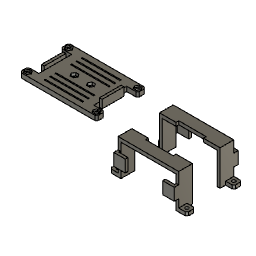
Bbox_lite_mount (Autodesk Fusion 360 design; units mm, degrees)
Autodesk Fusion 360 part; units mm, degrees
note: some values were not read from the file. Set by a fixed rule: which face or edge a step refers to.
sketch "Sketch1" plane through (0, 0, 0) normal (0, 0, 1) x (1, 0, 0)
  line L0 (0, 0) -> (100.25, 0)
  line L1 (100.25, 0) -> (100.25, -89.65)
  line L2 (100.25, -89.65) -> (0, -89.65)
  line L3 (0, -89.65) -> (0, 0)
  line L4 (100.25, 0) -> (105.25, 0)
  line L5 (105.25, 0) -> (105.25, -15)
  line L6 (105.25, -15) -> (100.25, -15)
  line L7 (100.25, -15) -> (100.25, 0)
  line L8 (105.25, 0) -> (120.25, 0)
  line L9 (120.25, 0) -> (120.25, -15)
  line L10 (120.25, -15) -> (105.25, -15)
  line L11 (105.25, -15) -> (105.25, 0)
  line L12 (100.25, -89.65) -> (105.25, -89.65)
  line L13 (105.25, -89.65) -> (105.25, -74.65)
  line L14 (105.25, -74.65) -> (100.25, -74.65)
  line L15 (100.25, -74.65) -> (100.25, -89.65)
  line L16 (105.25, -89.65) -> (120.25, -89.65)
  line L17 (120.25, -89.65) -> (120.25, -74.65)
  line L18 (120.25, -74.65) -> (105.25, -74.65)
  line L19 (105.25, -74.65) -> (105.25, -89.65)
  line L20 (0, 0) -> (-5, 0)
  line L21 (-5, 0) -> (-5, -15)
  line L22 (-5, -15) -> (0, -15)
  line L23 (0, -15) -> (0, 0)
  line L24 (0, -89.65) -> (-5, -89.65)
  line L25 (-5, -89.65) -> (-5, -74.65)
  line L26 (-5, -74.65) -> (0, -74.65)
  line L27 (0, -74.65) -> (0, -89.65)
  line L28 (-5, -74.65) -> (-19.7343, -74.65)
  line L29 (-19.7343, -74.65) -> (-19.7343, -89.65)
  line L30 (-19.7343, -89.65) -> (-5, -89.65)
  line L31 (-5, -89.65) -> (-5, -74.65)
  line L32 (-5, -15) -> (-20, -15)
  line L33 (-20, -15) -> (-20, 0)
  line L34 (-20, 0) -> (-5, 0)
  line L35 (-5, 0) -> (-5, -15)
  line L36 (105.25, -25) -> (100.25, -25)
  line L37 (100.25, -25) -> (100.25, -64.65)
  line L38 (100.25, -64.65) -> (105.25, -64.65)
  line L39 (105.25, -64.65) -> (105.25, -25)
  line L40 (0, -25) -> (0, -65)
  line L41 (-5, -25) -> (0, -25)
  line L42 (0, -25) -> (0, -64.65)
  line L43 (0, -64.65) -> (-5, -64.65)
  line L44 (-5, -64.65) -> (-5, -25)
  line L45 (109.6301, -12.6251) -> (115.6285, -12.7644)
  line L46 (115.6285, -12.7644) -> (118.7484, -7.6394)
  line L47 (118.7484, -7.6394) -> (115.8699, -2.3749)
  line L48 (115.8699, -2.3749) -> (109.8715, -2.2356)
  line L49 (109.8715, -2.2356) -> (106.7516, -7.3606)
  line L50 (106.7516, -7.3606) -> (109.6301, -12.6251)
  circle A0 centre (112.75, -7.5) radius 3.05
  line L51 (109.75, -87.3462) -> (115.75, -87.3462)
  line L52 (115.75, -87.3462) -> (118.75, -82.15)
  line L53 (118.75, -82.15) -> (115.75, -76.9538)
  line L54 (115.75, -76.9538) -> (109.75, -76.9538)
  line L55 (109.75, -76.9538) -> (106.75, -82.15)
  line L56 (106.75, -82.15) -> (109.75, -87.3462)
  line L57 (109.75, -87.3462) -> (115.75, -87.3462) construction
  circle A1 centre (112.75, -82.15) radius 3.05
  line L58 (-15.2555, -87.3338) -> (-9.2556, -87.3584)
  line L59 (-9.2556, -87.3584) -> (-6.2344, -82.1745)
  line L60 (-6.2344, -82.1745) -> (-9.2131, -76.9662)
  line L61 (-9.2131, -76.9662) -> (-15.213, -76.9416)
  line L62 (-15.213, -76.9416) -> (-18.2343, -82.1255)
  line L63 (-18.2343, -82.1255) -> (-15.2555, -87.3338)
  circle A2 centre (-12.2343, -82.15) radius 3.05
  line L64 (-15.5, -12.6962) -> (-9.5, -12.6962)
  line L65 (-9.5, -12.6962) -> (-6.5, -7.5)
  line L66 (-6.5, -7.5) -> (-9.5, -2.3038)
  line L67 (-9.5, -2.3038) -> (-15.5, -2.3038)
  line L68 (-15.5, -2.3038) -> (-18.5, -7.5)
  line L69 (-18.5, -7.5) -> (-15.5, -12.6962)
  line L70 (-15.5, -12.6962) -> (-15.4999, -12.6962) construction
  circle A3 centre (-12.5, -7.5) radius 3.05
  line L71 (15, -10) -> (85, -10)
  line L72 (85, -10) -> (85, -12)
  line L73 (85, -12) -> (15, -12)
  line L74 (15, -12) -> (15, -10)
  line L75 (15, -20) -> (85, -20)
  line L76 (85, -20) -> (85, -22)
  line L77 (85, -22) -> (15, -22)
  line L78 (15, -22) -> (15, -20)
  line L79 (15, -30) -> (85, -30)
  line L80 (85, -30) -> (85, -32)
  line L81 (85, -32) -> (15, -32)
  line L82 (15, -32) -> (15, -30)
  line L83 (15, -80) -> (85, -80)
  line L84 (85, -80) -> (85, -78)
  line L85 (85, -78) -> (15, -78)
  line L86 (15, -78) -> (15, -80)
  line L87 (15, -70) -> (85, -70)
  line L88 (85, -70) -> (85, -68)
  line L89 (85, -68) -> (15, -68)
  line L90 (15, -68) -> (15, -70)
  line L91 (15, -60) -> (85, -60)
  line L92 (85, -60) -> (85, -58)
  line L93 (85, -58) -> (15, -58)
  line L94 (15, -58) -> (15, -60)
  line L95 (50.125, -44.825) -> (0, -45)
  line L96 (50.125, -44.825) -> (100.25, -44.825)
  line L97 (32.125, -39.6812) -> (29.125, -44.8774)
  line L98 (29.125, -44.8774) -> (32.125, -50.0735)
  line L99 (32.125, -50.0735) -> (38.125, -50.0735)
  line L100 (38.125, -50.0735) -> (41.125, -44.8774)
  line L101 (41.125, -44.8774) -> (38.125, -39.6812)
  line L102 (38.125, -39.6812) -> (32.125, -39.6812)
  line L103 (62.125, -50.0212) -> (68.125, -50.0212)
  line L104 (68.125, -50.0212) -> (71.125, -44.825)
  line L105 (71.125, -44.825) -> (68.125, -39.6288)
  line L106 (68.125, -39.6288) -> (62.125, -39.6288)
  line L107 (62.125, -39.6288) -> (59.125, -44.825)
  line L108 (59.125, -44.825) -> (62.125, -50.0212)
  circle A4 centre (35.125, -44.8774) radius 3.05
  circle A5 centre (65.125, -44.825) radius 3.05
  point P0 (112.75, -7.5)
  point P1 (112.75, -82.15)
  point P2 (-12.2343, -82.15)
  point P3 (-12.5, -7.5)
  point P4 (35.125, -44.8774)
  point P5 (65.125, -44.825)
  dimension "d1" = 100.25
  dimension "d2" = 89.65
  dimension "d3" = 5
  dimension "d4" = 15
  dimension "d5" = 15
  dimension "d6" = 15
  dimension "d7" = 5
  dimension "d8" = 15
  dimension "d9" = 15
  dimension "d10" = 15
  dimension "d11" = 5
  dimension "d12" = 15
  dimension "d13" = 15
  dimension "d18" = 39.65
  dimension "d19" = 6
  dimension "d20" = 7.5
  dimension "d21" = 7.5
  dimension "d22" = 6.1
  dimension "d23" = 6
  dimension "d24" = 0
  dimension "d25" = 7.5
  dimension "d26" = 7.5
  dimension "d27" = 6.1
  dimension "d28" = 6
  dimension "d29" = 7.5
  dimension "d30" = 7.5
  dimension "d31" = 6.1
  dimension "d32" = 6
  dimension "d33" = 0
  dimension "d35" = 7.5
  dimension "d36" = 7.5
  dimension "d37" = 6.1
  dimension "d38" = 70
  dimension "d39" = 2
  dimension "d40" = 70
  dimension "d41" = 2
  dimension "d42" = 70
  dimension "d43" = 2
  dimension "d44" = 70
  dimension "d45" = 2
  dimension "d46" = 70
  dimension "d47" = 2
  dimension "d48" = 70
  dimension "d49" = 2
  dimension "d50" = 50.125
  dimension "d51" = 44.825
  dimension "d52" = 6
  dimension "d53" = 15
  dimension "d56" = 15
  dimension "d57" = 6.1
  dimension "d58" = 6.1
  constraint horizontal L0
  constraint vertical L1
  constraint horizontal L2
  constraint vertical L3
  constraint coincident L0.start L3.end
  constraint horizontal L4
  constraint vertical L5
  constraint horizontal L6
  constraint vertical L7
  constraint horizontal L8
  constraint vertical L9
  constraint horizontal L10
  constraint vertical L11
  constraint horizontal L12
  constraint vertical L13
  constraint horizontal L14
  constraint vertical L15
  constraint horizontal L16
  constraint vertical L17
  constraint horizontal L18
  constraint vertical L19
  constraint horizontal L20
  constraint vertical L21
  constraint horizontal L22
  constraint vertical L23
  constraint horizontal L24
  constraint vertical L25
  constraint horizontal L26
  constraint vertical L27
  constraint horizontal L28
  constraint vertical L29
  constraint horizontal L30
  constraint vertical L31
  constraint horizontal L32
  constraint vertical L33
  constraint horizontal L34
  constraint vertical L35
  constraint horizontal L36
  constraint vertical L37
  constraint horizontal L38
  constraint vertical L39
  constraint coincident L1 L37.end
  constraint vertical L40
  constraint coincident L3 L40.end
  constraint horizontal L41
  constraint vertical L42
  constraint horizontal L43
  constraint vertical L44
  constraint coincident P0 A0.centre
  constraint horizontal L57
  constraint coincident P1 A1.centre
  constraint coincident P2 A2.centre
  constraint horizontal L70
  constraint coincident P3 A3.centre
  constraint horizontal L71
  constraint vertical L72
  constraint horizontal L73
  constraint vertical L74
  constraint horizontal L75
  constraint vertical L76
  constraint horizontal L77
  constraint vertical L78
  constraint horizontal L79
  constraint vertical L80
  constraint horizontal L81
  constraint vertical L82
  constraint horizontal L83
  constraint vertical L84
  constraint horizontal L85
  constraint vertical L86
  constraint horizontal L87
  constraint vertical L88
  constraint horizontal L89
  constraint vertical L90
  constraint horizontal L91
  constraint vertical L92
  constraint horizontal L93
  constraint vertical L94
  constraint midpoint L40 L95.end
  constraint midpoint L37 L96.end
  constraint perpendicular L37 L96
  constraint coincident L95 P4
  constraint coincident L96 P5
  constraint coincident P4 A4.centre
  constraint coincident P5 A5.centre
  measures "d1" distance of L0.start L0.end
  measures "d2" distance of L0.start L2.end
  measures "d3" distance of L0.end L4.end
  measures "d4" distance of L0.end L6.end
  measures "d5" distance of L4.end L8.end
  measures "d6" distance of L4.end L5.end
  measures "d7" distance of L1.end L12.end
  measures "d8" distance of L1.end L14.end
  measures "d9" distance of L12.end L16.end
  measures "d10" distance of L12.end L13.end
  measures "d11" distance of L2.end L24.end
  measures "d12" distance of L2.end L26.end
  measures "d13" distance of L25.end L24.end
  measures "d18" distance of L41.start L43.end
  measures "d19" distance of L45.start L45.end
  measures "d20" distance of L10 P0
  measures "d21" distance of L9 P0
  measures "d22" diameter of A0
  measures "d23" distance of L51.start L51.end
  measures "d24" angle of L51 L57
  measures "d25" distance of L17 P1
  measures "d26" distance of L16 P1
  measures "d27" diameter of A1
  measures "d28" distance of L58.start L58.end
  measures "d29" distance of L29 P2
  measures "d30" distance of L30 P2
  measures "d31" diameter of A2
  measures "d32" distance of L64.start L64.end
  measures "d33" angle of L64 L70
  measures "d35" distance of L35 P3
  measures "d36" distance of L32 P3
  measures "d37" diameter of A3
  measures "d38" distance of L71.start L71.end
  measures "d39" distance of L71.start L73.end
  measures "d40" distance of L75.start L75.end
  measures "d41" distance of L75.start L77.end
  measures "d42" distance of L79.start L79.end
  measures "d43" distance of L79.start L81.end
  measures "d44" distance of L83.start L83.end
  measures "d45" distance of L83.start L85.end
  measures "d46" distance of L87.start L87.end
  measures "d47" distance of L87.start L89.end
  measures "d48" distance of L91.start L91.end
  measures "d49" distance of L91.start L93.end
  measures "d50" distance of L1 L95.start
  measures "d51" distance of L2 L95.start
  measures "d52" distance of L97.start L101.end
  measures "d53" horizontal distance of L95.start P4
  measures "d56" distance of L95.start P5
  measures "d57" diameter of A4
  measures "d58" diameter of A5
extrude "Extrude1" add sketch "Sketch1" along normal blind 8.35 contours L0 L1 L3 L7 L23 L37 L40 L42 L95 L96 L97 L98 L101 L102 L105 L106 L107 | L3 L20 L21 L22 L23 L35 | L1 L4 L5 L6 L7 L11 | L21 L32 L33 L34 L35 | L5 L8 L9 L10 L11 | L1 L2 L3 L15 L27 L37 L40 L42 L95 L96 L98 L99 L100 L101 L103 L104 L108 | L1 L12 L13 L14 L15 L19 | L3 L24 L25 L26 L27 L31 | L13 L16 L17 L18 L19 | L25 L28 L29 L30 L31 makes body 1
extrude "Extrude2" add sketch "Sketch1" along normal blind 15 contours L3 L40 L41 L42 L43 L44 | L1 L36 L37 L38 L39 bodies 1
extrude "Extrude3" add sketch "Sketch1" along normal blind 5.75 contours L45 L46 L47 L48 L49 L50 | L51 L52 L53 L54 L55 L56 | L58 L59 L60 L61 L62 L63 | L64 L65 L66 L67 L68 L69 bodies 1
extrude "Extrude4" add sketch "Sketch1" along normal blind 3.25 contours L95 L97 L98 L101 L102 A4 | L95 L98 L99 L100 L101 A4 | L96 L103 L104 L108 A5 | L96 L105 L106 L107 A5 bodies 1
chamfer "Chamfer1" distance 3 angle 45 8 edges at (120.25, -89.65, 4.175) (120.25, -74.65, 4.175) (120.25, -15, 4.175) (120.25, 0, 4.175) (-19.7343, -89.65, 4.175) (-19.7343, -74.65, 4.175) (-20, -15, 4.175) (-20, 0, 4.175) on bodies 1
sketch "Sketch2" plane through (0, 0, 0) normal (0, 0, 1) x (1, 0, 0)
  line L0 (175, 0) -> (275.25, 0)
  line L1 (275.25, 0) -> (275.25, -25)
  line L2 (275.25, -25) -> (175, -25)
  line L3 (175, -25) -> (175, 0)
  line L4 (175, 0) -> (170, 0)
  line L5 (170, 0) -> (170, -25)
  line L6 (170, -25) -> (175, -25)
  line L7 (175, -25) -> (175, 0)
  line L8 (275.25, 0) -> (280.25, 0)
  line L9 (280.25, 0) -> (280.25, -25)
  line L10 (280.25, -25) -> (275.25, -25)
  line L11 (275.25, -25) -> (275.25, 0)
  line L12 (200, -25) -> (250, -25)
  line L13 (250, -25) -> (250, -20)
  line L14 (250, -20) -> (200, -20)
  line L15 (200, -20) -> (200, -25)
  dimension "d68" = 100.25
  dimension "d69" = 25
  dimension "d70" = 5
  dimension "d71" = 5
  constraint horizontal L0
  constraint vertical L1
  constraint horizontal L2
  constraint vertical L3
  constraint horizontal L4
  constraint vertical L5
  constraint horizontal L6
  constraint vertical L7
  constraint horizontal L8
  constraint vertical L9
  constraint horizontal L10
  constraint vertical L11
  constraint horizontal L12
  constraint vertical L13
  constraint horizontal L14
  constraint vertical L15
  constraint coincident L2 L12.start
  measures "d68" distance of L0.start L0.end
  measures "d69" distance of L0.start L2.end
  measures "d70" distance of L0.start L4.end
  measures "d71" distance of L0.end L8.end
extrude "Extrude5" add sketch "Sketch2" along normal blind 6.35 separate body contours L0 L1 L2 L3 L7 L11 L13 L14 L15 | L3 L4 L5 L6 L7 | L1 L8 L9 L10 L11 makes body 2
extrude "Extrude6" add sketch "Sketch2" against normal blind 57.55 contours L3 L4 L5 L6 L7 | L1 L8 L9 L10 L11 bodies 2
sketch "Sketch3" plane through (280.25, 0, 0) normal (1, 0, 0) x (0, 1, 0)
  line L0 (0, -57.55) -> (0, 6.35)
  line L1 (0, 6.35) -> (-25, 6.35)
  line L2 (-25, 6.35) -> (-25, -57.55)
  line L3 (-25, -57.55) -> (0, -57.55)
  line L4 (0, -57.55) -> (-15, -57.55)
  line L5 (-15, -57.55) -> (-15, -51.2)
  line L6 (-15, -51.2) -> (0, -51.2)
  line L7 (0, -51.2) -> (0, -57.55)
  dimension "d76" = 15
  dimension "d77" = 6.35
  constraint horizontal L4
  constraint vertical L5
  constraint horizontal L6
  constraint vertical L7
  constraint coincident L0.start L3.end
  measures "d76" distance of L0.start L4.end
  measures "d77" distance of L0.start L6.end
extrude "Extrude7" add sketch "Sketch3" along normal blind 15 contours L0 L3 L4 L5 L6 L7 bodies 2
sketch "Sketch4" plane through (170, 0, 0) normal (-1, 0, 0) x (0, -1, 0)
  line L0 (25, -57.55) -> (25, 6.35)
  line L1 (25, 6.35) -> (0, 6.35)
  line L2 (0, 6.35) -> (0, -57.55)
  line L3 (0, -57.55) -> (25, -57.55)
  line L4 (0, -57.55) -> (15, -57.55)
  line L5 (15, -57.55) -> (15, -51.2)
  line L6 (15, -51.2) -> (0, -51.2)
  line L7 (0, -51.2) -> (0, -57.55)
  dimension "d80" = 15
  dimension "d81" = 6.35
  constraint horizontal L4
  constraint vertical L5
  constraint horizontal L6
  constraint vertical L7
  constraint coincident L2.end L3.start
  measures "d80" distance of L2.end L4.end
  measures "d81" distance of L2.end L6.end
extrude "Extrude8" add sketch "Sketch4" along normal blind 15 contours L2 L3 L4 L5 L6 L7 bodies 2
sketch "Sketch5" plane through (0, 0, -51.2) normal (0, 0, 1) x (-1, 0, 0)
  line L0 (-280.25, 0) -> (-280.25, 15)
  line L1 (-280.25, 15) -> (-295.25, 15)
  line L2 (-295.25, 15) -> (-295.25, 0)
  line L3 (-295.25, 0) -> (-280.25, 0)
  line L4 (-284.7018, 2.332) -> (-281.7503, 7.5558)
  line L5 (-281.7503, 7.5558) -> (-284.7985, 12.7238)
  line L6 (-284.7985, 12.7238) -> (-290.7982, 12.668)
  line L7 (-290.7982, 12.668) -> (-293.7497, 7.4442)
  line L8 (-293.7497, 7.4442) -> (-290.7015, 2.2762)
  line L9 (-290.7015, 2.2762) -> (-284.7018, 2.332)
  circle A0 centre (-287.75, 7.5) radius 3.05
  point P0 (-287.75, 7.5)
  dimension "d84" = 6
  dimension "d85" = 7.5
  dimension "d86" = 7.5
  dimension "d87" = 6.1
  constraint coincident P0 A0.centre
  measures "d84" distance of L4.start L8.end
  measures "d85" distance of L3 P0
  measures "d86" distance of L2 P0
  measures "d87" diameter of A0
sketch "Sketch6" plane through (0, 0, -57.55) normal (0, 0, -1) x (1, 0, 0)
  line L0 (280.25, 25) -> (275.25, 25)
  line L1 (275.25, 25) -> (275.25, 0)
  line L2 (275.25, 0) -> (295.25, 0)
  line L3 (295.25, 0) -> (295.25, 15)
  line L4 (295.25, 15) -> (280.25, 15)
  line L5 (280.25, 15) -> (280.25, 25)
  circle A0 centre (287.75, 7.5) radius 3.05
  line L6 (290.7982, 12.668) -> (293.7497, 7.4442)
  line L7 (293.7497, 7.4442) -> (290.7015, 2.2762)
  line L8 (290.7015, 2.2762) -> (284.7018, 2.332)
  line L9 (284.7018, 2.332) -> (281.7503, 7.5558)
  line L10 (281.7503, 7.5558) -> (284.7985, 12.7238)
  line L11 (284.7985, 12.7238) -> (290.7982, 12.668)
  point P0 (287.75, 7.5)
sketch "Sketch7" plane through (0, 0, -51.2) normal (0, 0, 1) x (-1, 0, 0)
  line L0 (-170, 15) -> (-170, 0)
  line L1 (-170, 0) -> (-155, 0)
  line L2 (-155, 0) -> (-155, 15)
  line L3 (-155, 15) -> (-170, 15)
  line L4 (-159.4638, 2.3249) -> (-156.5001, 7.5419)
  line L5 (-156.5001, 7.5419) -> (-159.5363, 12.717)
  line L6 (-159.5363, 12.717) -> (-165.5362, 12.6751)
  line L7 (-165.5362, 12.6751) -> (-168.4999, 7.4581)
  line L8 (-168.4999, 7.4581) -> (-165.4637, 2.283)
  line L9 (-165.4637, 2.283) -> (-159.4638, 2.3249)
  circle A0 centre (-162.5, 7.5) radius 3.05
  point P0 (-162.5, 7.5)
  dimension "d88" = 6
  dimension "d89" = 7.5
  dimension "d90" = 7.5
  dimension "d91" = 6.1
  constraint coincident P0 A0.centre
  measures "d88" distance of L4.start L8.end
  measures "d89" distance of L1 P0
  measures "d90" distance of L2 P0
  measures "d91" diameter of A0
sketch "Sketch8" plane through (0, 0, -57.55) normal (0, 0, -1) x (1, 0, 0)
  line L0 (175, 0) -> (175, 25)
  line L1 (175, 25) -> (170, 25)
  line L2 (170, 25) -> (170, 15)
  line L3 (170, 15) -> (155, 15)
  line L4 (155, 15) -> (155, 0)
  line L5 (155, 0) -> (175, 0)
  circle A0 centre (162.5, 7.5) radius 3.05
  line L6 (159.4638, 2.3249) -> (156.5001, 7.5419)
  line L7 (165.4637, 2.283) -> (159.4638, 2.3249)
  line L8 (168.4999, 7.4581) -> (165.4637, 2.283)
  line L9 (165.5362, 12.6751) -> (168.4999, 7.4581)
  line L10 (159.5363, 12.717) -> (165.5362, 12.6751)
  line L11 (156.5001, 7.5419) -> (159.5363, 12.717)
  point P0 (162.5, 7.5)
chamfer "Chamfer2" distance 3 angle 45 4 edges at (295.25, -15, -54.375) (295.25, 0, -54.375) (155, -15, -54.375) (155, 0, -54.375) on bodies 2
extrude "Extrude9" cut sketch "Sketch8" sketch "Sketch6" against normal blind 2.5 contours L6 L7 L8 L9 L10 L11 of sketch 2 contours L6 L7 L8 L9 L10 L11 bodies 2
extrude "Extrude10" cut 2 faces at (163.1505, -6.9273, -57.55) (288.2946, -8.1401, -57.55) along direction (0, 0, 1) blind 6.35 on bodies 2 bodies 2
sketch "Sketch9" plane through (175, 0, 0) normal (1, 0, 0) x (0, 1, 0)
  line L0 (0, 0) -> (-25, 0)
  line L1 (-25, 0) -> (-25, -57.55)
  line L2 (-25, -57.55) -> (0, -57.55)
  line L3 (0, -57.55) -> (0, 0)
  line L4 (-15, -51.2) -> (0, -51.2)
  line L5 (-15, -51.2) -> (-15, -57.55)
sketch "Sketch10" plane through (275.25, 0, 0) normal (-1, 0, 0) x (0, -1, 0)
  line L0 (25, 0) -> (0, 0)
  line L1 (0, 0) -> (0, -57.55)
  line L2 (0, -57.55) -> (25, -57.55)
  line L3 (25, -57.55) -> (25, 0)
  line L4 (0, -51.2) -> (15, -51.2)
  line L5 (15, -57.55) -> (15, -51.2)
sketch "Sketch11" plane through (0, 0, 0) normal (0, 1, 0) x (-1, 0, 0)
  line L0 (-158, -57.55) -> (-158, -51.2)
  line L1 (-158, -51.2) -> (-170, -51.2)
  line L2 (-170, -51.2) -> (-170, 6.35)
  line L3 (-170, 6.35) -> (-280.25, 6.35)
  line L4 (-280.25, 6.35) -> (-280.25, -51.2)
  line L5 (-280.25, -51.2) -> (-292.25, -51.2)
  line L6 (-292.25, -51.2) -> (-292.25, -57.55)
  line L7 (-292.25, -57.55) -> (-275.25, -57.55)
  line L8 (-275.25, -57.55) -> (-275.25, 0)
  line L9 (-275.25, 0) -> (-175, 0)
  line L10 (-175, 0) -> (-175, -57.55)
  line L11 (-175, -57.55) -> (-158, -57.55)
  line L12 (-280.25, -14.6) -> (-275.25, -14.6)
  line L13 (-275.25, -14.6) -> (-275.25, -36.6)
  line L14 (-275.25, -36.6) -> (-280.25, -36.6)
  line L15 (-280.25, -36.6) -> (-280.25, -14.6)
  line L16 (-275.25, 0) -> (-280.25, 0)
  line L17 (-280.25, -51.2) -> (-275.25, -51.2)
  line L18 (-175, -36.6) -> (-170, -36.6)
  line L19 (-170, -36.6) -> (-170, -14.6)
  line L20 (-170, -14.6) -> (-175, -14.6)
  line L21 (-175, -14.6) -> (-175, -36.6)
  line L22 (-175, 0) -> (-170, 0)
  line L23 (-170, -51.2) -> (-175, -51.2)
  dimension "d97" = 22
  dimension "d98" = 5
  dimension "d99" = 14.6
  dimension "d100" = 22
  dimension "d101" = 14.6
  constraint horizontal L12
  constraint vertical L13
  constraint horizontal L14
  constraint vertical L15
  constraint coincident L4 L12.start
  constraint coincident L8.end L9.start
  constraint coincident L4 L16.end
  constraint perpendicular L4 L16
  constraint coincident L4.end L5.start
  constraint perpendicular L8 L17
  constraint horizontal L18
  constraint vertical L19
  constraint horizontal L20
  constraint vertical L21
  constraint coincident L10 L18.start
  constraint coincident L9.end L10.start
  constraint coincident L2 L22.end
  constraint perpendicular L2 L22
  constraint coincident L1.end L2.start
  constraint coincident L10 L23.end
  constraint perpendicular L10 L23
  measures "d97" distance of L12.start L14.end
  measures "d98" distance of L4.end L17.end
  measures "d99" distance of L12 L16
  measures "d100" distance of L18.start L20.end
  measures "d101" distance of L20 L22
copy_body "CopyPasteBodies1" bodies 2 makes body 3
move_body "Move1" bodies 3 to x (-1, 0, 0) y (0, -1, 0) z (0, 0, 1) at (450, -100, 0)
extrude "Extrude11" add sketch "Sketch11" along normal blind 8.2 contours L2 L10 L18 L19 L20 L21 | L4 L8 L12 L13 L14 L15 bodies 2
sketch "Sketch12" plane through (175, 0, 0) normal (1, 0, 0) x (0, 1, 0)
  line L0 (0, 0) -> (-25, 0)
  line L1 (-25, 0) -> (-25, -57.55)
  line L2 (-25, -57.55) -> (0, -57.55)
  line L3 (0, -57.55) -> (0, -36.6)
  line L4 (0, -36.6) -> (8.2, -36.6)
  line L5 (8.2, -36.6) -> (8.2, -14.6)
  line L6 (8.2, -14.6) -> (0, -14.6)
  line L7 (0, -14.6) -> (0, 0)
  line L8 (8.2, -14.6) -> (3.2, -14.6)
  line L9 (3.2, -14.6) -> (3.2, -36.6)
  line L10 (3.2, -36.6) -> (8.2, -36.6)
  line L11 (8.2, -36.6) -> (8.2, -14.6)
  line L12 (3.2, -14.6) -> (0, -14.6)
  line L13 (0, -14.6) -> (0, -36.6)
  line L14 (0, -36.6) -> (3.2, -36.6)
  line L15 (3.2, -36.6) -> (3.2, -14.6)
  dimension "d104" = 5
  constraint horizontal L8
  constraint vertical L9
  constraint horizontal L10
  constraint vertical L11
  constraint coincident L5.end L6.start
  constraint horizontal L12
  constraint vertical L13
  constraint horizontal L14
  constraint vertical L15
  constraint coincident L3.end L4.start
  measures "d104" distance of L5.end L8.end
sketch "Sketch13" plane through (275.25, 0, 0) normal (-1, 0, 0) x (0, -1, 0)
  line L0 (25, 0) -> (0, 0)
  line L1 (0, 0) -> (0, -14.6)
  line L2 (0, -14.6) -> (-8.2, -14.6)
  line L3 (-8.2, -14.6) -> (-8.2, -36.6)
  line L4 (-8.2, -36.6) -> (0, -36.6)
  line L5 (0, -36.6) -> (0, -57.55)
  line L6 (0, -57.55) -> (25, -57.55)
  line L7 (25, -57.55) -> (25, 0)
  line L8 (-8.2, -14.6) -> (-3.2, -14.6)
  line L9 (-3.2, -14.6) -> (-3.2, -36.6)
  line L10 (-3.2, -36.6) -> (-8.2, -36.6)
  line L11 (-8.2, -36.6) -> (-8.2, -14.6)
  line L12 (-3.2, -14.6) -> (0, -14.6)
  line L13 (0, -14.6) -> (0, -36.6)
  line L14 (0, -36.6) -> (-3.2, -36.6)
  line L15 (-3.2, -36.6) -> (-3.2, -14.6)
  dimension "d105" = 5
  constraint horizontal L8
  constraint vertical L9
  constraint horizontal L10
  constraint vertical L11
  constraint coincident L2.end L3.start
  constraint horizontal L12
  constraint vertical L13
  constraint horizontal L14
  constraint vertical L15
  constraint coincident L4.end L5.start
  measures "d105" distance of L2.end L8.end
extrude "Extrude12" add sketch "Sketch13" along normal blind 20 contours L2 L3 L4 L8 L9 L10 L11 L15 bodies 2
extrude "Extrude13" add sketch "Sketch12" along normal blind 20 contours L4 L5 L6 L8 L9 L10 L11 L15 bodies 2
sketch "Sketch14" plane through (0, -100, 0) normal (0, -1, 0) x (1, 0, 0)
  line L0 (292, -57.55) -> (292, -51.2)
  line L1 (292, -51.2) -> (280, -51.2)
  line L2 (280, -51.2) -> (280, 6.35)
  line L3 (280, 6.35) -> (169.75, 6.35)
  line L4 (169.75, 6.35) -> (169.75, -51.2)
  line L5 (169.75, -51.2) -> (157.75, -51.2)
  line L6 (157.75, -51.2) -> (157.75, -57.55)
  line L7 (157.75, -57.55) -> (174.75, -57.55)
  line L8 (174.75, -57.55) -> (174.75, 0)
  line L9 (174.75, 0) -> (275, 0)
  line L10 (275, 0) -> (275, -57.55)
  line L11 (275, -57.55) -> (292, -57.55)
  line L12 (169.75, -14.6) -> (174.75, -14.6)
  line L13 (174.75, -14.6) -> (174.75, -36.6)
  line L14 (174.75, -36.6) -> (169.75, -36.6)
  line L15 (169.75, -36.6) -> (169.75, -14.6)
  line L16 (174.75, 0) -> (169.75, 0)
  line L17 (169.75, -51.2) -> (174.75, -51.2)
  line L18 (275, -14.6) -> (280, -14.6)
  line L19 (280, -14.6) -> (280, -36.6)
  line L20 (280, -36.6) -> (275, -36.6)
  line L21 (275, -36.6) -> (275, -14.6)
  line L22 (275, 0) -> (280, 0)
  line L23 (280, -51.2) -> (275, -51.2)
  dimension "d110" = 22
  dimension "d111" = 5
  dimension "d112" = 5
  dimension "d113" = 14.6
  dimension "d114" = 22
  dimension "d115" = 14.6
  constraint horizontal L12
  constraint vertical L13
  constraint horizontal L14
  constraint vertical L15
  constraint coincident L4 L12.start
  constraint coincident L8.end L9.start
  constraint perpendicular L4 L16
  constraint coincident L4.end L5.start
  constraint perpendicular L8 L17
  constraint horizontal L18
  constraint vertical L19
  constraint horizontal L20
  constraint vertical L21
  constraint coincident L10 L18.start
  constraint coincident L9.end L10.start
  constraint coincident L2 L22.end
  constraint perpendicular L2 L22
  constraint coincident L1.end L2.start
  constraint coincident L10 L23.end
  constraint perpendicular L10 L23
  measures "d110" distance of L12.start L14.end
  measures "d111" distance of L8.end L16.end
  measures "d112" distance of L4.end L17.end
  measures "d113" distance of L12 L16
  measures "d114" distance of L18.start L20.end
  measures "d115" distance of L18 L22
extrude "Extrude14" add sketch "Sketch14" along normal blind 8.1 contours L2 L10 L18 L19 L20 L21 | L4 L8 L12 L13 L14 L15 bodies 3
sketch "Sketch15" plane through (174.75, 0, 0) normal (1, 0, 0) x (0, 1, 0)
  line L0 (-75, 0) -> (-100, 0)
  line L1 (-100, 0) -> (-100, -14.6)
  line L2 (-100, -14.6) -> (-108.1, -14.6)
  line L3 (-108.1, -14.6) -> (-108.1, -36.6)
  line L4 (-108.1, -36.6) -> (-100, -36.6)
  line L5 (-100, -36.6) -> (-100, -57.55)
  line L6 (-100, -57.55) -> (-75, -57.55)
  line L7 (-75, -57.55) -> (-75, 0)
  line L8 (-108.1, -14.6) -> (-103.1, -14.6)
  line L9 (-103.1, -14.6) -> (-103.1, -36.6)
  line L10 (-103.1, -36.6) -> (-108.1, -36.6)
  line L11 (-108.1, -36.6) -> (-108.1, -14.6)
  line L12 (-103.1, -14.6) -> (-100, -14.6)
  line L13 (-100, -14.6) -> (-100, -36.6)
  line L14 (-100, -36.6) -> (-103.1, -36.6)
  line L15 (-103.1, -36.6) -> (-103.1, -14.6)
  dimension "d118" = 5
  constraint horizontal L8
  constraint vertical L9
  constraint horizontal L10
  constraint vertical L11
  constraint coincident L2.end L3.start
  constraint horizontal L12
  constraint vertical L13
  constraint horizontal L14
  constraint vertical L15
  constraint coincident L4.end L5.start
  measures "d118" distance of L2.end L8.end
sketch "Sketch16" plane through (275, 0, 0) normal (-1, 0, 0) x (0, -1, 0)
  line L0 (100, 0) -> (75, 0)
  line L1 (75, 0) -> (75, -57.55)
  line L2 (75, -57.55) -> (100, -57.55)
  line L3 (100, -57.55) -> (100, -36.6)
  line L4 (100, -36.6) -> (108.1, -36.6)
  line L5 (108.1, -36.6) -> (108.1, -14.6)
  line L6 (108.1, -14.6) -> (100, -14.6)
  line L7 (100, -14.6) -> (100, 0)
  line L8 (108.1, -14.6) -> (103.1, -14.6)
  line L9 (103.1, -14.6) -> (103.1, -36.6)
  line L10 (103.1, -36.6) -> (108.1, -36.6)
  line L11 (108.1, -36.6) -> (108.1, -14.6)
  line L12 (103.1, -14.6) -> (100, -14.6)
  line L13 (100, -14.6) -> (100, -36.6)
  line L14 (100, -36.6) -> (103.1, -36.6)
  line L15 (103.1, -36.6) -> (103.1, -14.6)
  dimension "d119" = 5
  constraint horizontal L8
  constraint vertical L9
  constraint horizontal L10
  constraint vertical L11
  constraint coincident L5.end L6.start
  constraint horizontal L12
  constraint vertical L13
  constraint horizontal L14
  constraint vertical L15
  constraint coincident L3.end L4.start
  measures "d119" distance of L5.end L8.end
extrude "Extrude15" add sketch "Sketch15" along normal blind 16 contours L2 L3 L4 L8 L9 L10 L11 L15 bodies 3
extrude "Extrude16" add sketch "Sketch16" along normal blind 16 contours L4 L5 L6 L8 L9 L10 L11 L15 bodies 3
extrude "Extrude17" cut sketch "Sketch15" against normal blind 0.925 contours L2 L4 L9 L12 L13 L14 L15 bodies 3
extrude "Extrude18" cut sketch "Sketch16" against normal blind 0.925 contours L4 L6 L9 L12 L13 L14 L15 bodies 3
extrude "Extrude19" cut sketch "Sketch13" against normal blind 0.925 contours L2 L4 L9 L12 L13 L14 L15 bodies 2
extrude "Extrude20" cut sketch "Sketch12" against normal blind 0.925 contours L4 L6 L9 L12 L13 L14 L15 bodies 2
equation "d74 = -51.20 mm - 6.35 mm"
equation "d102 = 2.7 mm + 0.5 mm + 5 mm"
equation "d116 = 2.6 mm + 0.5 mm + 5 mm"
